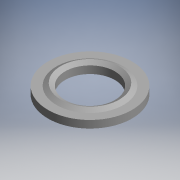
# Autodesk Inventor part: 1451339 M10-NBR-10x16.9x1.5
Saved by Autodesk Inventor 2017.3 (Build 213256000, 256)
## iProperties
Part Number: 1451339 M10-NBR-10x16.9x1.5
Material: Generic
Catalog Web Link: www.cadenas.de
Description: NBR-sealing ring
Vendor: FESTO
Document SubType Name: Modeling
Designer: partserver
Manufacturer: FESTO
Mass: 0.250586 g
Surface Area: 4.38071 cm^2
Volume: 0.250586 cm^3
Density: 1 g/cm^3
Appearance: PSOLRGB-192-192-192
Category: PARTsolutions
Company: FESTO
Title: 1451339 M10-NBR-10x16.9x1.5
Author: Cadenas PARTsolutions
Comments: sealing ring
PSOL_IDENT_0: {$CADENAS_DATA\23d-libs\festo\parts\e\eamm\parts\eamm_u_nbr.prj},192 {VTYP=3D},{NB=1451339 M10-NBR-1
PSOL_IDENT_1: 0x16.9x1.5},{LINA=1451339 M10-NBR-10x16.9x1.5},{NN=NBR},{DATE=27.10.2020 09:44:40},{GEOMDATE=08.01.2
PSOL_IDENT_2: 020 14:15:00},{VERSION=},{LINEID=530},{WBVAR=},{WBNUMERIC=}  {NB=1451339 M10-NBR-10x16.9x1.5},{LINA=
PSOL_IDENT_3: 1451339 M10-NBR-10x16.9x1.5},{KT=DUMMY},{TNR=1451339},{TYP=M10-NBR-10x16.9x1.5},{FG=M10},{D1=16.900}
PSOL_IDENT_4: ,{D2=10.000},{S1=1.500},{S2=2.500}
NB: 1451339 M10-NBR-10x16.9x1.5
NN: NBR
NT: sealing ring
NBSYN: $TNR. $TYP.
LINA: 1451339 M10-NBR-10x16.9x1.5
CATALOG: Festo
TNR: 1451339
TYP: M10-NBR-10x16.9x1.5
FG: M10
D1: 16.9
D2: 10
S1: 1.5
S2: 2.5
SUPPLIER: FESTO
ARTICLENO: 1451339 M10-NBR-10x16.9x1.5
BOMINFO: 1451339 M10-NBR-10x16.9x1.5
CREATOR: CADENAS GmbH
Autodesk Inventor part; units mm, degrees
sketch "Sketch_1" plane through (0, 0, 0) normal (1, 0, 0) x (0, 1, 0)
  line L0 (0, 0) -> (0, 2.5)
  line L1 (5.866, 2.5) -> (5, 2)
  line L2 (5, 2) -> (5, 0.5)
  line L3 (5, 0.5) -> (5.866, 0)
  line L4 (5.866, 0) -> (6.7321, 0.5)
  line L5 (6.7321, 0.5) -> (8.45, 0.5)
  line L6 (8.45, 0.5) -> (8.45, 2)
  line L7 (8.45, 2) -> (6.7321, 2)
  line L8 (6.7321, 2) -> (5.866, 2.5)
  constraints: 18 end point
revolve "Revolution1" add sketch "Sketch_1" angle 360 about axis through (0, 0, 0) along (0, 0, -1)
ref_plane "ANBAU1_XY" through (0, 0, 0) normal (0, 0, 1) x (1, 0, 0)
ref_plane "ANBAU1_YZ" through (0, 0, 0) normal (1, 0, 0) x (0, 1, 0)
ref_plane "ANBAU1_ZX" through (0, 0, 0) normal (0, 1, 0) x (0, 0, 1)
ref_plane "ANBAU2_XY" through (0, 0, 2.5) normal (0, 0, 1) x (1, 0, 0)
ref_plane "ANBAU2_YZ" through (0, 0, 2.5) normal (1, 0, 0) x (0, 1, 0)
ref_plane "ANBAU2_ZX" through (0, 0, 2.5) normal (0, 1, 0) x (0, 0, 1)
body "Solid1"
